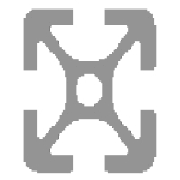
# Autodesk Inventor part: COTS_ARMA_AR3701_20x20_Alu_Extr_00000002
Saved by Autodesk Inventor 2026.1 (Build 301233000, 233)
## iProperties
_CCFamilyDisplayName: AR3701 profil 20x20 _frame - AR3701 profil 20x20
_FrameMemberDoc: Frame Member File
_Version: 25.0.0
_GetPNFromCC: 1
Created: 2016-06-20
Part Number: COTS_ARMA_AR3701_20x20_Alu_Extr_00000002
Material: Aluminium 6061-AHC
Description: AR3701 profil 20x20
Document SubType Name: Modeling
Standard: AR3701 profil 20x20
Designer: Andrzej
Standard Revision: AR3701 profil 20x20
Manufacturer: AR3701 profil 20x20
Standards Organization: AR3701 profil 20x20
Language: pl-PL
Size Designation: (Bez nazwy 1)
Categories: <MemberInstance><Categories><Category DisplayName="Kształtowniki konstrukcyjne" InternalName="089c4875-fa83-4c05-b084-43b9cc11f5ed" Mnemonic="GRDR"><CategoryParameter DisplayName="Masa na jednostkę długości" InternalName="0bb95a10-148f-4027-a459-38d7b056702a" Mnemonic="shpmass"/><CategoryParameter DisplayName="Powierzchnia przekroju" InternalName="1ff91680-64b0-4202-b9a3-7fd3f94bba3b" Mnemonic="secarea"/><CategoryParameter DisplayName="Promień obrotu (x)" InternalName="25778675-03e9-40c1-b6a8-4a9ed693320d" Mnemonic="gyrradx"/><CategoryParameter DisplayName="Moduł sztywności skrętnej" InternalName="26c1ec35-5026-4c63-ad0a-751cf684a536" Mnemonic="torrigmod"/><CategoryParameter DisplayName="Odległość środka ciężkości X-X" InternalName="26c9bdb8-9c79-4b4f-a92e-8e197583c9c4" Mnemonic="grcendistX"/><CategoryParameter DisplayName="ID elementu typowego" InternalName="340afe4f-75d7-48d3-ab7d-943f3c3da468" Mnemonic="LegacyMemberID"/><CategoryParameter DisplayName="Długość podstawowa" InternalName="42e34263-8f20-4d0e-ad48-bf1385b87c24" Mnemonic="shplen"/><CategoryParameter DisplayName="Moment bezwładności (y)" InternalName="4b9f58ea-bced-460e-81ea-3d29ca5a49e3" Mnemonic="inermomy"/><CategoryParameter DisplayName="Moment bezwładności (x)" InternalName="4cd780bc-73d7-43ac-917a-579e5cbd684d" Mnemonic="inermomx"/><CategoryParameter DisplayName="Niestandardowy punkt podstawowy" InternalName="4f1d1b73-316d-484b-a3df-9cbabb16eb77" Mnemonic="shpBasePoint"/><CategoryParameter DisplayName="Wysokość kształtki" InternalName="50274e7d-5ac0-4796-92cb-c59e54983c67" Mnemonic="shpheig"/><CategoryParameter DisplayName="Moduł wytrzymałości przekroju (y)" InternalName="59eaa5e9-d227-48dc-b6c1-6920f96e0f95" Mnemonic="secmody"/><CategoryParameter DisplayName="Oznaczenie fragmentu" InternalName="5a64d034-428d-49c8-ba32-7619764de20f" Mnemonic="shpdes"/><CategoryParameter DisplayName="Moduł wytrzymałości przekroju (x)" InternalName="72cfad18-cf51-4ed4-aaa7-c6b224f8419f" Mnemonic="secmodx"/><CategoryParameter DisplayName="Moduł wytrzymałości przekroju na skręcanie" InternalName="7c55a8dc-8844-49f9-a867-cc677b30ec9a" Mnemonic="torsecmod"/><CategoryParameter DisplayName="Szerokość kształtki" InternalName="7c717d54-a18f-4666-b4d4-573cce22c62c" Mnemonic="shpwdth"/><CategoryParameter DisplayName="Grubość drugiej kształtki" InternalName="9251a8e1-85fd-4e47-af99-afdb762317d9" Mnemonic="shpthick2"/><CategoryParameter DisplayName="Złącze zatwierdzone" InternalName="9c666724-f362-4ea7-ac62-f6a007de5c69" Mnemonic="shpFGAuto"/><CategoryParameter DisplayName="Odległość środka ciężkości Y-Y" InternalName="bcc4fb17-7af4-436a-8f8c-d0aa3b0248c5" Mnemonic="grcendistY"/><CategoryParameter DisplayName="Promień obrotu (y)" InternalName="bfa18ebe-1636-4dbe-8d42-b263e0b73184" Mnemonic="gyrrady"/><CategoryParameter DisplayName="Grubość kształtki" InternalName="d109cf76-8eb4-42fc-9800-4409734adc67" Mnemonic="shpthick"/><CategoryParameter DisplayName="Współczynnik przesunięcia w wyniku ścinania" InternalName="de4c90c6-aaa8-468f-a335-6737b311b5d3" Mnemonic="shdispc"/><Category DisplayName="Inne" InternalName="f02205ff-2390-476f-921c-0b3185f88e84" Mnemonic="OTHSHP"><CategoryParameter DisplayName="Moment bezwładności (y)" InternalName="044c654e-f649-48ac-84cc-650a29ae31ca" Mnemonic="inermomy"/><CategoryParameter DisplayName="Grubość kształtki" InternalName="12b1a788-9233-48fd-a933-2df8ff42b15f" Mnemonic="shpthick"/><CategoryParameter DisplayName="Masa na jednostkę długości" InternalName="2fd289d6-9394-4d2d-97e6-6659d7d4551d" Mnemonic="shpmass"/><CategoryParameter DisplayName="Promień obrotu (y)" InternalName="743e1dfe-1bba-408b-b985-cf752b207386" Mnemonic="gyrrady"/><CategoryParameter DisplayName="Moduł wytrzymałości przekroju (y)" InternalName="88b8bff9-a616-4028-93d5-ed4f79680d13" Mnemonic="secmody"/><CategoryParameter DisplayName="Powierzchnia przekroju" InternalName="c46ecdf8-b6eb-4db9-8b25-30258930c1e3" Mnemonic="secarea"/><CategoryParameter DisplayName="Moduł wytrzymałości przekroju (x)" InternalName="cac70804-9d39-43bb-be17-56ea1f39a6c2" Mnemonic="secmodx"/><CategoryParameter DisplayName="Moment bezwładności (x)" InternalName="ec6737bc-264f-43ed-b0bd-f6d410c2718d" Mnemonic="inermomx"/><CategoryParameter DisplayName="Promień obrotu (x)" InternalName="ee72c61e-565e-4fd6-b448-66e1e1abcb7e" Mnemonic="gyrradx"/></Category></Category><Category DisplayName="TypDanych" InternalName="23b78d0f-2648-40c6-8793-ca6db495c9e8" Mnemonic="DATATYPE"><CategoryParameter DisplayName="NazwaWyświetlana" InternalName="05415f3d-3907-474b-a020-eb9d644f4cf3" Mnemonic="DISPLAYNAME"/><CategoryParameter DisplayName="Standardowe" InternalName="0c0a119c-1e12-4c84-803f-101930972f5e" Mnemonic="STANDARD"/><CategoryParameter DisplayName="Opis" InternalName="13903e3d-64b1-4950-80da-f627842ea37f" Mnemonic="DESCRIPTION"/><CategoryParameter DisplayName="Oznaczenie" InternalName="2675968c-4ce5-49e0-a4f5-552d29089031" Mnemonic="DESIGNATION"/><CategoryParameter DisplayName="Wiersz domyślny" InternalName="2af9ec52-faaa-4026-b378-f9fa4afca842" Mnemonic="DEFAULTROW"/><CategoryParameter DisplayName="Nazwa folderu" InternalName="3f06958e-8713-4116-9be7-ed6184ecc97b" Mnemonic="FOLDERNAME"/><CategoryParameter DisplayName="Wskazówki do poprawek" InternalName="45a75005-10b1-4dfc-8d6d-dfe629f0b93c" Mnemonic="REVISIONGUID"/><CategoryParameter DisplayName="Nazwa pliku" InternalName="8b46a4cc-9585-4fed-90c3-899f57e09a73" Mnemonic="FILENAME"/><CategoryParameter DisplayName="OrgStd" InternalName="8f5914e1-4693-403f-8ab5-d37768198c9d" Mnemonic="STDSORG"/><CategoryParameter DisplayName="Wersja rodziny" InternalName="914462f6-6e19-4b14-ba84-155b9680b1d0" Mnemonic="FAMILYREVISION"/><CategoryParameter DisplayName="Poprawka standardowa" InternalName="91d5a463-65c2-4fde-b823-3b7fea5e8e17" Mnemonic="STANDARDREVISION"/><CategoryParameter DisplayName="Zmiana elementu" InternalName="a65d44b9-392f-4f4f-857b-e4b3d54996fe" Mnemonic="MEMBERREVISION"/><CategoryParameter DisplayName="FormatKlipu" InternalName="bc51e27b-3422-4e78-93ef-cec197ddf230" Mnemonic="CLIPFORMAT"/><CategoryParameter DisplayName="Producent" InternalName="cd6c7a72-a28a-4e50-99a9-2c7f4e13e5ad" Mnemonic="MANUFACTURER"/><CategoryParameter DisplayName="NazwaWewnętrzna" InternalName="cf1d0246-76d9-4b4a-8305-fa0409afb5c1" Mnemonic="INTERNALNAME"/><CategoryParameter DisplayName="CzyMetryczne" InternalName="e2385c5b-1ea4-4823-96a8-8de651266ec3" Mnemonic="ISMETRIC"/><Category DisplayName="Część" InternalName="c0e0b642-3bcb-4cc8-9e80-f96d35c4afa4" Mnemonic="PART"><CategoryParameter DisplayName="Numer części" InternalName="016b6077-bfbe-49bd-92c9-d8d59c39c941" Mnemonic="PARTNUMBER"/><CategoryParameter DisplayName="Numer katalogowy" InternalName="4dba7c1c-e26c-444e-836c-b08b433409a8" Mnemonic="STOCKNUMBER"/><CategoryParameter DisplayName="Klucz - materiał" InternalName="5c9a8adb-dd2b-4535-b97f-0a94a95fe41f" Mnemonic="MATERIALKEY"/><CategoryParameter DisplayName="Materiał" InternalName="818a152a-d3c3-49ca-80ee-df7d91421b8e" Mnemonic="MATERIAL"/></Category></Category></Categories><FamilyTemplate Id="AR3701 profil 20x20 _frame"><FamilyTemplateParameters><FamilyTemplateParameter ObjectType="kModelParameterObject" ValueType="xs:double" Id="12" ObjectReferenceKey="Length"/><FamilyTemplateParameter ObjectType="kPartComponentDefinitionObject" ValueType="xs:string" Id="23" SubObjectId="Material"/><FamilyTemplateParameter ObjectType="kPropertyObject" ValueType="xs:string" Id="26" ObjectReferenceKey="{32853F0F-3444-11d1-9E93-0060B03C1CA6}" SubObjectId="5"/><FamilyTemplateParameter ObjectType="kPropertyObject" ValueType="xs:string" Id="27" ObjectReferenceKey="{32853F0F-3444-11d1-9E93-0060B03C1CA6}" SubObjectId="52"/></FamilyTemplateParameters></FamilyTemplate><CategoryParameterMap><ParamToTemplateMap><ParamToTemplate CategoryParameter="//CategoryParameter[@InternalName='cf1d0246-76d9-4b4a-8305-fa0409afb5c1']" ConstantValue="fc560555-dec5-4fde-a77b-daa6e84102e2"/><ParamToTemplate CategoryParameter="//CategoryParameter[@InternalName='45a75005-10b1-4dfc-8d6d-dfe629f0b93c']" ConstantValue="50e74c9d-fffe-42dc-9045-91c60e27ea6e"/><ParamToTemplate CategoryParameter="//CategoryParameter[@InternalName='3f06958e-8713-4116-9be7-ed6184ecc97b']" ConstantValue="AR3701 profil 20x20 _frame"/><ParamToTemplate CategoryParameter="//CategoryParameter[@InternalName='8f5914e1-4693-403f-8ab5-d37768198c9d']" ConstantValue="AR3701 profil 20x20"/><ParamToTemplate CategoryParameter="//CategoryParameter[@InternalName='0c0a119c-1e12-4c84-803f-101930972f5e']" ConstantValue="AR3701 profil 20x20"/><ParamToTemplate CategoryParameter="//CategoryParameter[@InternalName='91d5a463-65c2-4fde-b823-3b7fea5e8e17']" ConstantValue="AR3701 profil 20x20"/><ParamToTemplate CategoryParameter="//CategoryParameter[@InternalName='cd6c7a72-a28a-4e50-99a9-2c7f4e13e5ad']" ConstantValue="AR3701 profil 20x20"/><ParamToTemplate CategoryParameter="//CategoryParameter[@InternalName='13903e3d-64b1-4950-80da-f627842ea37f']" ConstantValue="AR3701 profil 20x20"/><ParamToTemplate CategoryParameter="//CategoryParameter[@InternalName='05415f3d-3907-474b-a020-eb9d644f4cf3']" ConstantValue="AR3701 profil 20x20 _frame"/><ParamToTemplate CategoryParameter="//CategoryParameter[@InternalName='914462f6-6e19-4b14-ba84-155b9680b1d0']" ConstantValue="11"/><ParamToTemplate CategoryParameter="//CategoryParameter[@InternalName='bc51e27b-3422-4e78-93ef-cec197ddf230']" ConstantValue="CF_INVENTOR.STDPARTS"/><ParamToTemplate CategoryParameter="//CategoryParameter[@InternalName='e2385c5b-1ea4-4823-96a8-8de651266ec3']" ConstantValue="true"/><ParamToTemplate CategoryParameter="//CategoryParameter[@InternalName='2af9ec52-faaa-4026-b378-f9fa4afca842']" ConstantValue="1"/><ParamToTemplate CategoryParameter="//CategoryParameter[@InternalName='9c666724-f362-4ea7-ac62-f6a007de5c69']" ConstantValue="1"/><ParamToTemplate CategoryParameter="//CategoryParameter[@InternalName='8b46a4cc-9585-4fed-90c3-899f57e09a73']" ConstantValue="1"/><ParamToTemplate CategoryParameter="//CategoryParameter[@InternalName='a65d44b9-392f-4f4f-857b-e4b3d54996fe']" ConstantValue="a11ffdaf-82d9-49db-ab9f-7690424d2dab"/><ParamToTemplate CategoryParameter="//CategoryParameter[@InternalName='a65d44b9-392f-4f4f-857b-e4b3d54996fe']" ConstantValue="a11ffdaf-82d9-49db-ab9f-7690424d2dab"/><ParamToTemplate CategoryParameter="//CategoryParameter[@InternalName='2675968c-4ce5-49e0-a4f5-552d29089031']" TemplateParameter="27"/><ParamToTemplate CategoryParameter="//CategoryParameter[@InternalName='42e34263-8f20-4d0e-ad48-bf1385b87c24']" TemplateParameter="12"/><ParamToTemplate CategoryParameter="//CategoryParameter[@InternalName='818a152a-d3c3-49ca-80ee-df7d91421b8e']" TemplateParameter="23"/><ParamToTemplate CategoryParameter="//CategoryParameter[@InternalName='016b6077-bfbe-49bd-92c9-d8d59c39c941']" TemplateParameter="26"/></ParamToTemplateMap></CategoryParameterMap></MemberInstance>
Density: 2.7 g/cm^3
Appearance: Aluminium - ciemne
Mass: 181.581 g
Surface Area: 690.51 cm^2
Volume: 67.2521 cm^3
G_L: 390,000 mm
G_W: 20,000 mm
G_H: 20,000 mm
+C9085904-FD8B-4B82-934A-45C53E89B29B+CUTDETAIL1: Wytnij
+1FF90E21-268E-469C-8C12-FE1E20183E62+CUTDETAIL2: Wytnij
IsCustomPart: 1
Author: Andrzej
Autodesk Inventor part; units mm, degrees
ref_plane "Płaszczyzna początkowa" through (0, 0, 20) normal (0, 0, 1) x (1, 0, 0)
ref_plane "Płaszczyzna końcowa" through (0, 0, 410) normal (0, 0, 1) x (1, 0, 0)
sketch "Szkic" plane through (0, 0, 0) normal (0, 0, 1) x (1, 0, 0)
  arc A0 (8, -10) -> (10, -8) centre (8, -8) ccw
  line L0 (10, -8) -> (10, -3)
  arc A1 (10, -3) -> (9.5, -2.5) centre (9.5, -3) ccw
  line L1 (9.5, -2.5) -> (8.4, -2.5)
  arc A2 (8.4, -2.5) -> (8.2, -2.7) centre (8.4, -2.7) ccw
  line L2 (8.2, -2.7) -> (8.2, -5.3428)
  arc A3 (6.9197, -5.8732) -> (8.2, -5.3428) centre (7.45, -5.3428) ccw
  line L3 (6.9197, -5.8732) -> (4.3987, -3.3522)
  arc A4 (3.52, -1.2308) -> (4.3987, -3.3522) centre (6.52, -1.2308) ccw
  line L4 (3.52, -1.2308) -> (3.52, 1.2308)
  arc A5 (4.3987, 3.3522) -> (3.52, 1.2308) centre (6.52, 1.2308) ccw
  line L5 (4.3987, 3.3522) -> (6.9197, 5.8732)
  arc A6 (8.2, 5.3428) -> (6.9197, 5.8732) centre (7.45, 5.3428) ccw
  line L6 (8.2, 5.3428) -> (8.2, 2.7)
  arc A7 (8.2, 2.7) -> (8.4, 2.5) centre (8.4, 2.7) ccw
  line L7 (8.4, 2.5) -> (9.5, 2.5)
  arc A8 (9.5, 2.5) -> (10, 3) centre (9.5, 3) ccw
  line L8 (10, 3) -> (10, 8)
  arc A9 (10, 8) -> (8, 10) centre (8, 8) ccw
  line L9 (8, 10) -> (3, 10)
  arc A10 (3, 10) -> (2.5, 9.5) centre (3, 9.5) ccw
  line L10 (2.5, 9.5) -> (2.5, 8.4)
  arc A11 (2.5, 8.4) -> (2.7, 8.2) centre (2.7, 8.4) ccw
  line L11 (2.7, 8.2) -> (5.3428, 8.2)
  arc A12 (5.8732, 6.9197) -> (5.3428, 8.2) centre (5.3428, 7.45) ccw
  line L12 (5.8732, 6.9197) -> (3.3522, 4.3987)
  arc A13 (1.2308, 3.52) -> (3.3522, 4.3987) centre (1.2308, 6.52) ccw
  line L13 (1.2308, 3.52) -> (-1.2308, 3.52)
  arc A14 (-3.3522, 4.3987) -> (-1.2308, 3.52) centre (-1.2308, 6.52) ccw
  line L14 (-3.3522, 4.3987) -> (-5.8732, 6.9197)
  arc A15 (-5.3428, 8.2) -> (-5.8732, 6.9197) centre (-5.3428, 7.45) ccw
  line L15 (-5.3428, 8.2) -> (-2.7, 8.2)
  arc A16 (-2.7, 8.2) -> (-2.5, 8.4) centre (-2.7, 8.4) ccw
  line L16 (-2.5, 8.4) -> (-2.5, 9.5)
  arc A17 (-2.5, 9.5) -> (-3, 10) centre (-3, 9.5) ccw
  line L17 (-3, 10) -> (-8, 10)
  arc A18 (-8, 10) -> (-10, 8) centre (-8, 8) ccw
  line L18 (-10, 8) -> (-10, 3)
  arc A19 (-10, 3) -> (-9.5, 2.5) centre (-9.5, 3) ccw
  line L19 (-9.5, 2.5) -> (-8.4, 2.5)
  arc A20 (-8.4, 2.5) -> (-8.2, 2.7) centre (-8.4, 2.7) ccw
  line L20 (-8.2, 2.7) -> (-8.2, 5.3428)
  arc A21 (-6.9197, 5.8732) -> (-8.2, 5.3428) centre (-7.45, 5.3428) ccw
  line L21 (-6.9197, 5.8732) -> (-4.3987, 3.3522)
  arc A22 (-3.52, 1.2308) -> (-4.3987, 3.3522) centre (-6.52, 1.2308) ccw
  line L22 (-3.52, 1.2308) -> (-3.52, -1.2308)
  arc A23 (-4.3987, -3.3522) -> (-3.52, -1.2308) centre (-6.52, -1.2308) ccw
  line L23 (-4.3987, -3.3522) -> (-6.9197, -5.8732)
  arc A24 (-8.2, -5.3428) -> (-6.9197, -5.8732) centre (-7.45, -5.3428) ccw
  line L24 (-8.2, -5.3428) -> (-8.2, -2.7)
  arc A25 (-8.2, -2.7) -> (-8.4, -2.5) centre (-8.4, -2.7) ccw
  line L25 (-8.4, -2.5) -> (-9.5, -2.5)
  arc A26 (-9.5, -2.5) -> (-10, -3) centre (-9.5, -3) ccw
  line L26 (-10, -3) -> (-10, -8)
  arc A27 (-10, -8) -> (-8, -10) centre (-8, -8) ccw
  line L27 (-8, -10) -> (-3, -10)
  arc A28 (-3, -10) -> (-2.5, -9.5) centre (-3, -9.5) ccw
  line L28 (-2.5, -9.5) -> (-2.5, -8.4)
  arc A29 (-2.5, -8.4) -> (-2.7, -8.2) centre (-2.7, -8.4) ccw
  line L29 (-2.7, -8.2) -> (-5.3428, -8.2)
  arc A30 (-5.8732, -6.9197) -> (-5.3428, -8.2) centre (-5.3428, -7.45) ccw
  line L30 (-5.8732, -6.9197) -> (-3.3522, -4.3987)
  arc A31 (-1.2308, -3.52) -> (-3.3522, -4.3987) centre (-1.2308, -6.52) ccw
  line L31 (-1.2308, -3.52) -> (1.2308, -3.52)
  arc A32 (3.3522, -4.3987) -> (1.2308, -3.52) centre (1.2308, -6.52) ccw
  line L32 (3.3522, -4.3987) -> (5.8732, -6.9197)
  arc A33 (5.3428, -8.2) -> (5.8732, -6.9197) centre (5.3428, -7.45) ccw
  line L33 (5.3428, -8.2) -> (2.7, -8.2)
  arc A34 (2.7, -8.2) -> (2.5, -8.4) centre (2.7, -8.4) ccw
  line L34 (2.5, -8.4) -> (2.5, -9.5)
  arc A35 (2.5, -9.5) -> (3, -10) centre (3, -9.5) ccw
  line L35 (3, -10) -> (8, -10)
  circle A36 centre (0, 0) radius 2.15
  point P0 (10, -10)
  constraints: 72 end point, 72 point on circle, 37 centre point
extrude "Bryła" add sketch "Szkic" along normal up to surface (390 mm away) from surface at 20
sketch "Szkic4" plane through (0, 0, 0) normal (0, 0, 1) x (1, 0, 0)
  line L0 (0, 0) -> (10, 0)
ref_plane "Płaszczyzna konstrukcyjna4" through (0, 0, 0) normal (0, -1, 0) x (1, 0, 0)
sketch "Szkic5" plane through (0, 0, 0) normal (0, -1, 0) x (1, 0, 0)
  line L0 (-2, 20) -> (12, 20)
  line L1 (-2, 410) -> (12, 410)
  dimension "d7" = 390
  measures "d7" distance between parallel lines of L0 L1
ref_plane "Płaszczyzna konstrukcyjna5" through (3, 450, 410) normal (0, 0, 1) x (1, 0, 0)
split "Podział1" plane through (3, 450, 410) removes the side toward (0, 0, 1)
ref_plane "Płaszczyzna konstrukcyjna6" through (8, 440, 20) normal (0, 0, -1) x (-1, 0, 0)
split "Podział2" plane through (8, 440, 20) removes the side toward (0, 0, -1)
equation "\"G_L\" = d7"
